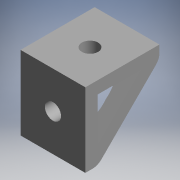
# Autodesk Inventor part: 4332
Saved by Autodesk Inventor 2017.3 (Build 213256000, 256)
## iProperties
Part Number: 4332
Material: Generic
Catalog Web Link: www.cadenas.de
Description: 4132, 4332, 4132-Black, 4332-Black-Joining Plates - 2 Hole Inside Gusset Corner Bracket
Vendor: 8020
Document SubType Name: Modeling
Designer: partserver
Manufacturer: 8020
Mass: 19.1831 g
Surface Area: 80.5939 cm^2
Volume: 19.1831 cm^3
Density: 1 g/cm^3
Appearance: PSOLRGB-191-191-191
Category: PARTsolutions
Company: 8020
Title: 4332
Author: Cadenas PARTsolutions
Comments: Joining Plates - 2 Hole Inside Gusset Corner Bracket
PSOL_IDENT_0: {$CADENAS_DATA\23d-libs\8020\inch\joining_plates\4132.prj},176 {VTYP=3D},{NB=4332},{LINA=4332},{NN=4
PSOL_IDENT_1: 132, 4332, 4132-Black, 4332-Black},{DATE=31.07.2020 09:21:18},{GEOMDATE=10.07.2017 17:29:09},{VERSIO
PSOL_IDENT_2: N=},{LINEID=20},{WBVAR=},{WBNUMERIC=}  {NB=4332},{LINA=4332},{KT=DUMMY},{PN=4332},{A=1.312},{B=1.500
PSOL_IDENT_3: },{C=1.500},{E=0.500},{F=0.328},{W=.125},{A1=0.6560},{C2=0.750},{D1=0.250},{C3=0.750},{COLOR=.75,.75
PSOL_IDENT_4: ,.75}
NB: 4332
NN: 4132, 4332, 4132-Black, 4332-Black
NT: Joining Plates - 2 Hole Inside Gusset Corner Bracket
NBSYN: $PN.
LINA: 4332
CATALOG: 80/20
PN: 4332
A: 1.312
B: 1.5
C: 1.5
W: .125
SUPPLIER: 8020
ARTICLENO: 4332
BOMINFO: 4332
CREATOR: CADENAS GmbH
Autodesk Inventor part; units mm, degrees
ref_plane "YZ Plane" through (0, 0, 0) normal (1, 0, 0) x (0, 1, 0)
ref_plane "XZ Plane" through (0, 0, 0) normal (0, 1, 0) x (-1, 0, 0)
ref_plane "XY Plane" through (0, 0, 0) normal (0, 0, 1) x (1, 0, 0)
sketch "Sketch_1" plane through (0, 0, 0) normal (1, 0, 0) x (0, 1, 0)
  line L0 (3.7197, 38.1) -> (0, 38.1)
  line L1 (0, 38.1) -> (0, 0)
  line L2 (0, 0) -> (38.1, 0)
  line L3 (38.1, 0) -> (38.1, 3.7197)
  arc A0 (38.1, 3.7197) -> (36.2401, 8.2099) centre (31.75, 3.7197) ccw
  line L4 (36.2401, 8.2099) -> (8.2099, 36.2401)
  arc A1 (8.2099, 36.2401) -> (3.7197, 38.1) centre (3.7197, 31.75) ccw
  line L5 (6.35, 29.1197) -> (6.35, 6.35)
  line L6 (6.35, 6.35) -> (29.1197, 6.35)
  line L7 (29.1197, 6.35) -> (6.35, 29.1197)
  constraints: 16 end point, 4 point on circle, 2 centre point
extrude "Extrusion1" add sketch "Sketch_1" along normal mid plane 33.3248
sketch "Sketch2" plane through (-16.6624, 0, 0) normal (0, -1, 0) x (1, 0, 0)
  point P0 (16.6624, 19.05)
hole "Hole1" at (0, 0, 19.05) direction (0, 1, 0) diameter 8.3312 depth 6.35
sketch "Sketch3" plane through (16.6624, 38.1, 0) normal (0, 0, -1) x (-1, 0, 0)
  point P0 (16.6624, -19.05)
hole "Hole2" at (0, 19.05, 0) direction (0, 0, 1) diameter 8.3312 depth 6.35
sketch "Sketch_4" plane through (0, 0, 38.1) normal (0, 0, 1) x (1, 0, 0)
  circle A0 centre (0, 19.05) radius 9.525
  constraints: 1 centre point
extrude "Extrusion2" cut sketch "Sketch_4" against normal blind 31.75
sketch "Sketch_5" plane through (0, 38.1, 0) normal (0, 1, 0) x (1, 0, 0)
  circle A0 centre (0, -19.05) radius 9.525
  constraints: 1 centre point
extrude "Extrusion3" cut sketch "Sketch_5" against normal blind 31.75
body "Solid1"
